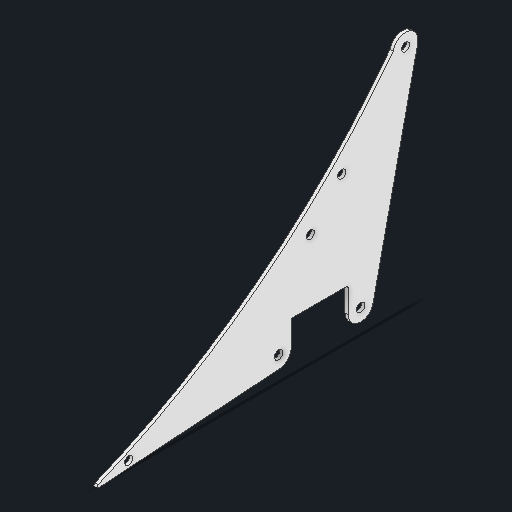
# Autodesk Inventor part: Ramp V2
Saved by Autodesk Inventor 2025.1 (Build 291241000, 241)
## iProperties
Created: 2024-10-13
Part Number: Ramp V2
Material: Acetal Resin, White
Document SubType Name: Sheet Metal
Designer: Averey Ku
Density: 1.425 g/cm^3
Appearance: Smooth - White
Mass: 12.8393 g
Surface Area: 122.133 cm^2
Volume: 9.01001 cm^3
Flat Pattern Width: 13.2826 cm
Flat Pattern Length: 15.3579 cm
Flat Pattern Area: 203.992 cm^2
Sheet Metal Rule: Default_mm
Sheet Metal Width: 5.229 in
Sheet Metal Length: 6.046 in
Sheet Metal Area: 31.619 in^2
Author: Averey Ku
Autodesk Inventor part; units mm, degrees
ref_plane "YZ Plane" through (0, 0, 0) normal (1, 0, 0) x (0, 1, 0)
ref_plane "XZ Plane" through (0, 0, 0) normal (0, 1, 0) x (-1, 0, 0)
ref_plane "XY Plane" through (0, 0, 0) normal (0, 0, 1) x (1, 0, 0)
sketch "main" plane through (0, 0, 0) normal (0, 0, 1) x (1, 0, 0)
  circle A0 centre (-198.1135, 49.9495) radius 2.1844
  circle A1 centre (-95.8324, -13.8772) radius 2.1
  arc A2 (-99.5351, -19.036) -> (-94.63, -7.6421) centre (-95.8324, -13.8772) ccw
  arc A3 (-204.4481, 49.5075) -> (-198.1135, 43.5995) centre (-198.1135, 49.9495) ccw
  line L0 (-210.7981, 140.5057) -> (-204.4481, 49.5075)
  arc A4 (-209.271, 140.8599) -> (-94.63, -7.6421) centre (115.0165, 272.7027) ccw
  circle A5 centre (-206.375, 125.4125) radius 2.0828
  line L1 (-198.1135, 43.5995) -> (-186.2072, 43.5995)
  arc A6 (-209.271, 140.8599) -> (-210.7981, 140.5057) centre (-210.0063, 140.561) ccw
  circle A7 centre (-135.2274, 18.1995) radius 2.0828
  line L2 (-185.4135, 15.8183) -> (-185.4135, 42.8058)
  line L3 (-198.1135, 15.0245) -> (-186.2072, 15.0245)
  arc A8 (-185.4135, 42.8058) -> (-186.2072, 43.5995) centre (-186.2072, 42.8058) ccw
  arc A9 (-186.2072, 15.0245) -> (-185.4135, 15.8183) centre (-186.2072, 15.8183) ccw
  line L4 (-199.4808, 2.4735) -> (-97.1997, -20.0783)
  circle A10 centre (-198.1135, 8.6745) radius 2.1848
  arc A11 (-198.1135, 15.0245) -> (-199.4808, 2.4735) centre (-198.1135, 8.6745) ccw
  point P0 (1.1251, 9.7944)
  point P1 (-211.1526, 145.5863)
  point P2 (-191.7635, 49.9495)
  dimension "d7" = 12.7
  dimension "d8" = 4.1656
  dimension "d9" = 6.35
  dimension "d11" = 0.7937
  dimension "d13" = 4.1656
  dimension "d16" = 0.7937
  dimension "d19" = 26.9875
  dimension "d20" = 0
  dimension "d21" = 6.35
  dimension "d24" = 6.35
  measures "d7" diameter of A3
  measures "d8" diameter of A5
  measures "d9" radius of A2
  measures "d11" radius of A6
  measures "d13" diameter of A7
  measures "d16" radius of A8
  measures "d19" distance of A9.centre A8.centre
  measures "d20" vertical distance of point (-191.763, 49.95) A0.centre
  measures "d21" distance of point (-191.763, 49.95) A0.centre
  measures "d24" horizontal distance of L0.end L0.start
sketch "Sketch1" plane through (0, 0, 0) normal (1, 0, 0) x (0, 1, 0)
  circle A0 centre (44.45, -15.875) radius 2.0955
  circle A1 centre (0, 0) radius 2.1844
  circle A2 centre (102.2811, -63.8268) radius 2.1
  arc A3 (98.5784, -68.9855) -> (103.4835, -57.5917) centre (102.2811, -63.8268) ccw
  arc A4 (-6.3346, -0.442) -> (0, -6.35) centre (0, 0) ccw
  line L0 (-12.6846, 90.5562) -> (-6.3346, -0.442)
  arc A5 (-11.1575, 90.9104) -> (103.4835, -57.5917) centre (313.1299, 222.7532) ccw
  circle A6 centre (-8.2615, 75.463) radius 2.0828
  line L1 (0, -6.35) -> (11.9063, -6.35)
  arc A7 (-11.1575, 90.9104) -> (-12.6846, 90.5562) centre (-11.8928, 90.6114) ccw
  circle A8 centre (62.8861, -31.75) radius 2.0828
  line L2 (12.7, -34.1313) -> (12.7, -7.1438)
  line L3 (0, -34.925) -> (11.9063, -34.925)
  arc A9 (12.7, -7.1438) -> (11.9063, -6.35) centre (11.9063, -7.1437) ccw
  arc A10 (11.9063, -34.925) -> (12.7, -34.1313) centre (11.9063, -34.1313) ccw
  line L4 (-1.3673, -47.4761) -> (100.9138, -70.0278)
  circle A11 centre (0, -41.275) radius 2.1848
  arc A12 (0, -34.925) -> (-1.3673, -47.4761) centre (0, -41.275) ccw
  dimension "d18" = 4.191
  constraints: 1 centre point, 1 other
  measures "d18" diameter of A0
extrude "Extrusion1" add sketch "Sketch1" along normal blind 1.5875
equation "\"BendRadius\" = Thickness"
equation "\"BendReliefWidth\" = Thickness"
equation "\"BendReliefDepth\" = 0.5 * Thickness"
equation "\"CornerReliefSize\" = 4 * Thickness"
equation "\"MinimumRemnant\" = 2 * Thickness"
equation "\"TransitionRadius\" = BendRadius"
equation "\"JacobiRadiusSize\" = BendRadius"
equation "\"GapSize\" = Thickness"
equation "\"Thickness\" = 1.5875"
body "Solid1"
